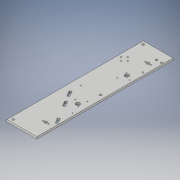
# Autodesk Inventor part: ChassisOutide10
Saved by Autodesk Inventor 2019 (Build 230136000, 136)
## iProperties
Created: 2019-10-11
Part Number: ChassisOutide10
Material: Generic
Document SubType Name: Modeling
Designer: shrey
Density: 1 g/cm^3
Appearance: Default
Author: shrey
Autodesk Inventor part; units mm, degrees
ref_plane "YZ Plane" through (0, 0, 0) normal (1, 0, 0) x (0, 1, 0)
ref_plane "XZ Plane" through (0, 0, 0) normal (0, 1, 0) x (-1, 0, 0)
ref_plane "XY Plane" through (0, 0, 0) normal (0, 0, 1) x (1, 0, 0)
sketch "Sketch1" plane through (0, 0, 0) normal (0, 1, 0) x (-1, 0, 0)
  line L0 (44.45, 203.2) -> (-44.45, 203.2)
  line L1 (-44.45, 203.2) -> (-44.45, -203.2)
  line L2 (-44.45, -203.2) -> (44.45, -203.2)
  line L3 (44.45, -203.2) -> (44.45, 203.2)
  line L4 (44.45, 203.2) -> (-44.45, -203.2) construction
  line L5 (-44.45, 203.2) -> (-20.955, 203.2)
  line L6 (-20.955, 203.2) -> (-20.955, 88.9) construction
  line L7 (-44.45, 88.9) -> (-44.45, 203.2)
  line L8 (44.45, 203.2) -> (44.45, 111.6492)
  line L9 (44.45, 203.2) -> (44.45, 38.1)
  line L10 (44.45, 38.1) -> (22.225, 38.1) construction
  line L11 (0, 203.2) -> (-66.675, 203.2)
  line L12 (-66.675, 203.2) -> (-66.675, 88.9) construction
  line L13 (-66.675, 203.2) -> (-66.675, 209.55) construction
  line L14 (-20.955, 114.3) -> (-20.955, 152.4) construction
  circle A0 centre (-20.955, 152.4) radius 8.001 construction
  circle A1 centre (-20.955, 152.4) radius 4.0005
  circle A2 centre (-20.955, 160.401) radius 1.85
  line L15 (17.145, 152.4) -> (-20.955, 152.4) construction
  circle A3 centre (-28.956, 152.4) radius 1.85
  line L16 (-20.955, 190.5) -> (-20.955, 152.4) construction
  circle A4 centre (-20.955, 144.399) radius 1.85
  line L17 (-59.055, 152.4) -> (-20.955, 152.4) construction
  circle A5 centre (-12.954, 152.4) radius 1.85
  line L18 (44.45, 0) -> (-44.45, 0) construction
  line L19 (32.5679, 18.912) -> (22.7595, 35.2429)
  line L20 (22.7595, 35.2429) -> (17.8553, 43.4083) construction
  line L21 (15.6729, 53.2085) -> (25.4813, 36.8776)
  line L22 (25.4813, 36.8776) -> (20.0377, 33.6081)
  line L23 (20.0377, 33.6081) -> (10.2292, 49.939)
  line L24 (10.2292, 49.939) -> (15.6729, 53.2085)
  line L25 (15.6729, 53.2085) -> (20.0377, 33.6081) construction
  line L26 (25.4813, 36.8776) -> (10.2292, 49.939) construction
  circle A6 centre (-20.955, -152.4) radius 4.0005
  circle A7 centre (-28.956, -152.4) radius 1.85
  circle A8 centre (-12.954, -152.4) radius 1.85
  line L27 (-44.45, 88.9) -> (-44.45, 12.7)
  line L28 (44.45, 203.2) -> (34.925, 203.2)
  line L29 (34.925, 203.2) -> (34.925, 193.675) construction
  line L30 (34.925, 193.675) -> (44.45, 193.675) construction
  line L31 (44.45, 193.675) -> (44.45, 203.2)
  circle A9 centre (34.925, 193.675) radius 3.175
  circle A10 centre (-31.75, 0) radius 3.175
  circle A11 centre (34.925, -193.675) radius 3.175
  line L32 (-44.45, 0) -> (-19.455, 0) construction
  line L33 (-16.28, -76.0639) -> (-22.63, -76.0639) construction
  line L34 (44.45, -203.2) -> (25.4, -203.2)
  line L35 (25.4, -203.2) -> (25.4, -128.2) construction
  line L36 (25.4, -128.2) -> (44.45, -128.2) construction
  line L37 (44.45, -128.2) -> (44.45, -203.2)
  circle A12 centre (25.4, -128.2) radius 6.35 construction
  circle A13 centre (25.4, -128.2) radius 9.779 construction
  circle A14 centre (15.621, -128.2) radius 1.778
  circle A15 centre (25.4, -128.2) radius 6.35 construction
  circle A16 centre (25.4, -128.2) radius 9.779 construction
  line L38 (100.4, -128.2) -> (25.4, -128.2) construction
  line L39 (25.4, -128.2) -> (25.4, -109.15) construction
  circle A17 centre (25.4, -137.979) radius 1.778
  circle A18 centre (25.4, -128.2) radius 6.35 construction
  circle A19 centre (25.4, -128.2) radius 9.779 construction
  line L40 (25.4, -53.2) -> (25.4, -128.2) construction
  line L41 (25.4, -128.2) -> (6.35, -128.2) construction
  circle A20 centre (35.179, -128.2) radius 1.778
  circle A21 centre (25.4, -128.2) radius 6.35 construction
  circle A22 centre (25.4, -128.2) radius 9.779 construction
  line L42 (-49.6, -128.2) -> (25.4, -128.2) construction
  line L43 (25.4, -128.2) -> (25.4, -147.25) construction
  circle A23 centre (25.4, -118.421) radius 1.778
  line L44 (21.8541, 5.2236) -> (22.225, 38.1) construction
  line L45 (-66.675, 209.55) -> (-66.675, 184.15)
  circle A24 centre (21.8541, 5.2236) radius 1.27
  circle A25 centre (21.8541, 5.2236) radius 12.7 construction
  line L46 (-9.3876, 82.6008) -> (-3.944, 85.8702)
  line L47 (-3.944, 85.8702) -> (5.8645, 69.5394)
  line L48 (0.4208, 66.2699) -> (-9.3876, 82.6008)
  line L49 (5.8645, 69.5394) -> (0.4208, 66.2699)
  line L50 (-29.0044, 115.2625) -> (-23.5608, 118.532)
  line L51 (-23.5608, 118.532) -> (-13.7524, 102.2011)
  line L52 (-19.196, 98.9316) -> (-29.0044, 115.2625)
  line L53 (-13.7524, 102.2011) -> (-19.196, 98.9316)
  line L54 (-20.955, 152.4) -> (-20.955, 104.775) construction
  circle A26 centre (-20.955, 152.4) radius 31.75 construction
  line L55 (-20.955, 104.775) -> (-20.955, 57.15) construction
  circle A27 centre (-20.955, -152.4) radius 30.48 construction
  line L56 (5.8645, 69.5394) -> (-36.6387, 140.3065) construction
  line L57 (-36.6387, 140.3065) -> (-26.8303, 123.9756)
  line L58 (-26.8303, 123.9756) -> (-32.2739, 120.7061)
  line L59 (-32.2739, 120.7061) -> (-42.0823, 137.037)
  line L60 (-42.0823, 137.037) -> (-36.6387, 140.3065)
  line L61 (-44.45, -128.1042) -> (-44.45, 88.9)
  circle A28 centre (-37.019, 88.9) radius 1.27
  line L62 (44.45, 203.2) -> (39.7485, 203.2)
  line L63 (39.7485, 203.2) -> (39.7485, 140.2644) construction
  line L64 (39.7485, 140.2644) -> (44.45, 140.2644) construction
  line L65 (44.45, 140.2644) -> (44.45, 203.2)
  line L66 (44.45, 203.2) -> (6.6345, 203.2)
  line L67 (6.6345, 203.2) -> (6.6345, 195.3768) construction
  line L68 (6.6345, 195.3768) -> (44.45, 195.3768) construction
  line L69 (44.45, 195.3768) -> (44.45, 203.2)
  line L70 (-44.45, -203.2) -> (-31.75, -203.2)
  line L71 (-44.45, -181.4027) -> (-44.45, -203.2)
  circle A29 centre (-20.955, 152.4) radius 50.8 construction
  line L72 (-49.719, 101.6) -> (-49.719, 76.2) construction
  circle A30 centre (-37.019, -121.0813) radius 2.413
  line L73 (-24.319, -108.3813) -> (-49.719, -108.3813) construction
  line L74 (-49.719, -108.3813) -> (-49.719, -133.7813) construction
  line L75 (-49.719, -133.7813) -> (-24.319, -133.7813) construction
  line L76 (-24.319, -133.7813) -> (-24.319, -108.3813) construction
  line L77 (-24.319, -108.3813) -> (-49.719, -133.7813) construction
  line L78 (-49.719, -108.3813) -> (-24.319, -133.7813) construction
  line L79 (-20.955, 152.4) -> (-20.955, 57.15) construction
  circle A31 centre (-20.955, 57.15) radius 5.969
  line L80 (-20.955, 57.15) -> (-20.955, 50.038) construction
  circle A32 centre (-20.955, 50.038) radius 15.494 construction
  circle A33 centre (-20.955, 50.038) radius 18.542 construction
  line L81 (-20.955, 50.038) -> (-36.449, 50.038) construction
  circle A34 centre (-36.449, 50.038) radius 1.27
  line L82 (-20.955, 50.038) -> (-28.702, 36.6198) construction
  circle A35 centre (-28.702, 36.6198) radius 1.27
  line L83 (-20.955, 50.038) -> (-13.208, 36.6198) construction
  circle A36 centre (-13.208, 36.6198) radius 1.27
  line L84 (-20.955, 50.038) -> (-5.461, 50.038) construction
  circle A37 centre (-5.461, 50.038) radius 1.27
  line L85 (-20.955, 50.038) -> (-13.208, 63.4562) construction
  circle A38 centre (-13.208, 63.4562) radius 1.27
  line L86 (-20.955, 50.038) -> (-28.702, 63.4562) construction
  circle A39 centre (-28.702, 63.4562) radius 1.27
  line L87 (-20.955, -152.4) -> (-20.955, -88.9) construction
  circle A40 centre (-20.955, -88.9) radius 5.969
  line L88 (-20.955, -88.9) -> (-20.955, -81.788) construction
  circle A41 centre (-20.955, -81.788) radius 15.494 construction
  line L89 (-20.955, -81.788) -> (-36.449, -81.788) construction
  circle A42 centre (-36.449, -81.788) radius 1.27
  circle A43 centre (-28.702, -95.2062) radius 1.27
  circle A44 centre (-13.208, -95.2062) radius 1.27
  circle A45 centre (-5.461, -81.788) radius 1.27
  circle A46 centre (-13.208, -68.3698) radius 1.27
  circle A47 centre (-28.702, -68.3698) radius 1.27
  circle A48 centre (-20.955, -81.788) radius 18.542 construction
  line L90 (-31.75, -173.862) -> (-39.7198, -173.862) construction
  circle A49 centre (-39.7198, -173.862) radius 3.048
  line L91 (-39.7198, -173.862) -> (-24.6385, -173.862) construction
  circle A50 centre (-24.6385, -173.862) radius 3.048
  point P0 (0, 0)
  dimension "d19" = 16.002
  dimension "d74" = 19.558
  dimension "d182" = 30.988
  dimension "d192" = 30.988
  dimension "d0" = 88.9
  dimension "d1" = 406.4
  dimension "d5" = 165.1
  dimension "d10" = 6.35
  dimension "d18" = 38.1
  dimension "d20" = 8.001
  dimension "d21" = 3.7
  dimension "d24" = 360
  dimension "d33" = 9.525
  dimension "d34" = 6.35
  dimension "d50" = 9.525
  dimension "d51" = 9.525
  dimension "d52" = 6.35
  dimension "d54" = 6.35
  dimension "d71" = 75
  dimension "d72" = 19.05
  dimension "d73" = 12.7
  dimension "d75" = 3.556
  dimension "d78" = 360
  dimension "d84" = 25.4
  dimension "d85" = 2.54
  dimension "d86" = 25.4
  dimension "d87" = 19.05
  dimension "d90" = 38.1
  dimension "d110" = 47.625
  dimension "d118" = 63.5
  dimension "d137" = 60.96
  dimension "d140" = 82.55
  dimension "d141" = 19.05
  dimension "d142" = 6.35
  dimension "d149" = 2.54
  dimension "d150" = 4.7015
  dimension "d151" = 62.9356
  dimension "d153" = 37.8155
  dimension "d154" = 7.8232
  dimension "d166" = 101.6
  dimension "d169" = 25.4
  dimension "d171" = 4.826
  dimension "d172" = 25.4
  dimension "d173" = 25.4
  dimension "d180" = 11.938
  dimension "d181" = 7.112
  dimension "d183" = 37.084
  dimension "d184" = 2.54
  dimension "d187" = 360
  dimension "d189" = 63.5
  dimension "d190" = 11.938
  dimension "d191" = 7.112
  dimension "d193" = 2.54
  dimension "d196" = 360
  dimension "d198" = 37.084
  dimension "d206" = 6.096
  dimension "d207" = 15.0813
  dimension "d208" = 6.096
  constraints: 184 end point, 44 centre point, 33 coincident, 18 parallel, 14 horizontal, 11 point on line, 9 perpendicular, 8 midpoint, 4 horizontal alignment, 4 symmetric about line, 4 vertical, 3 vertical alignment, 1 collinear, 143 other
  measures "d0" distance of L1.end L2.end
  measures "d1" distance of L0.end L1.end
  measures "d5" distance of L0.start L9.end
  measures "d10" distance of L11.end L13.end
  measures "d18" distance of L14.start L14.end
  measures "d20" diameter of A1
  measures "d21" diameter of A2
  measures "d33" distance of L20.start L20.end
  measures "d34" distance of L21.end L22.end
  measures "d50" distance of L29.end L30.end
  measures "d51" distance of L28.end L29.end
  measures "d52" diameter of A9
  measures "d54" diameter of A10
  measures "d71" distance of L34.end L35.end
  measures "d72" distance of L35.end L36.end
  measures "d73" diameter of A12
  measures "d75" diameter of A14
  measures "d84" distance of L13.end L45.end
  measures "d85" diameter of A24
  measures "d86" diameter of A25
  measures "d87" distance of L19.start L19.end
  measures "d90" distance of L23.end L46.start
  measures "d110" distance of L17.end L54.end
  measures "d118" diameter of A26
  measures "d137" diameter of A27
  measures "d140" distance of L47.end L56.end
  measures "d141" distance of L56.end L57.end
  measures "d142" distance of L57.end L58.end
  measures "d149" diameter of A28
  measures "d150" distance of L64.end L63.end
  measures "d151" distance of L63.end L62.end
  measures "d153" distance of L68.end L67.end
  measures "d154" distance of L67.end L66.end
  measures "d166" diameter of A29
  measures "d169" distance of L72.end L72.start
  measures "d171" diameter of A30
  measures "d172" distance of L75.end L74.end
  measures "d173" distance of L74.end L73.end
  measures "d180" diameter of A31
  measures "d181" distance of L80.start L80.end
  measures "d183" diameter of A33
  measures "d184" diameter of A34
  measures "d189" distance of L87.start L87.end
  measures "d190" diameter of A40
  measures "d191" distance of L88.start L88.end
  measures "d193" diameter of A42
  measures "d198" diameter of A48
  measures "d206" diameter of A49
  measures "d207" distance of L91.start L91.end
  measures "d208" diameter of A50
extrude "Extrusion16" add sketch "Sketch1" along normal blind 6.35 contours L3 L2 L1 L0 | A2 | A4 | L50 L51 L53 L52 | A34 | A36 | A38 | A43 | A45 | A47
body "Solid16"
